Autodesk Fusion 360 part; units mm, degrees
(part 2 of 2)
extrude "Foro_M2_5_barretta_Destra_01" cut sketch "Schizzo2 (11)" along normal blind 3 bodies 12 in component "08_Barrette_removibili_M2_5_SG90_Destra"
ref_plane "Piano di lavoro3" through (63.5, 0, 0) normal (1, 0, 0) x (0, 1, 0) in component "08_Barrette_removibili_M2_5_SG90_Destra"
sketch "Schizzo3 (9)" plane through (63.5, 0, 0) normal (1, 0, 0) x (0, 0, -1) in component "08_Barrette_removibili_M2_5_SG90_Destra"
  line L0 (-68.4, 2.7) -> (-81.6, 2.7)
  line L1 (-81.6, 2.7) -> (-81.6, 13.5)
  line L2 (-81.6, 13.5) -> (-68.4, 13.5)
  line L3 (-68.4, 13.5) -> (-68.4, 2.7)
extrude "Estrusione_Barretta_Destra_02" add sketch "Schizzo3 (9)" along normal blind 3 separate body makes body 13 in component "08_Barrette_removibili_M2_5_SG90_Destra"
ref_plane "Piano di lavoro4" through (63.5, 0, 0) normal (1, 0, 0) x (0, 1, 0) in component "08_Barrette_removibili_M2_5_SG90_Destra"
sketch "Schizzo4 (8)" plane through (63.5, 0, 0) normal (1, 0, 0) x (0, 0, -1) in component "08_Barrette_removibili_M2_5_SG90_Destra"
  circle A0 centre (-75, 12.25) radius 1.35
extrude "Foro_M2_5_barretta_Destra_02" cut sketch "Schizzo4 (8)" along normal blind 3 bodies 13 in component "08_Barrette_removibili_M2_5_SG90_Destra"
ref_plane "Piano di lavoro1" through (0, 0, 73) normal (0, 0, 1) x (1, 0, 0) in component "09_Torretta_parte_mobile_elevazione"
sketch "Schizzo1 (13)" plane through (0, 0, 73) normal (0, 0, 1) x (1, 0, 0) in component "09_Torretta_parte_mobile_elevazione"
  line L0 (-34, -20) -> (34, -20)
  line L1 (34, -20) -> (34, 50)
  line L2 (34, 50) -> (-34, 50)
  line L3 (-34, 50) -> (-34, -20)
extrude "Estrusione_Piastra_culla_mobile" add sketch "Schizzo1 (13)" along normal blind 4 separate body makes body 14 in component "09_Torretta_parte_mobile_elevazione"
sketch "Schizzo2 (12)" plane through (0, 0, 73) normal (0, 0, 1) x (1, 0, 0) in component "09_Torretta_parte_mobile_elevazione"
  line L0 (-3, -17) -> (3, -17)
  line L1 (3, -17) -> (3, -13)
  line L2 (3, -13) -> (-3, -13)
  line L3 (-3, -13) -> (-3, -17)
extrude "Passaggio_6x4_connettore_cannone_sotto_culla" cut sketch "Schizzo2 (12)" along normal blind 4 bodies 14 in component "09_Torretta_parte_mobile_elevazione"
sketch "Schizzo3 (10)" plane through (0, 0, 73) normal (0, 0, 1) x (1, 0, 0) in component "09_Torretta_parte_mobile_elevazione"
  circle A0 centre (-20, -5) radius 1.75
extrude "Foro_fissaggio_PCB_cannone_01" cut sketch "Schizzo3 (10)" along normal blind 4 bodies 14 in component "09_Torretta_parte_mobile_elevazione"
sketch "Schizzo4 (9)" plane through (0, 0, 73) normal (0, 0, 1) x (1, 0, 0) in component "09_Torretta_parte_mobile_elevazione"
  line L0 (-17.1, -3.3257) -> (-20, -1.6514)
  line L1 (-20, -1.6514) -> (-22.9, -3.3257)
  line L2 (-22.9, -3.3257) -> (-22.9, -6.6743)
  line L3 (-22.9, -6.6743) -> (-20, -8.3486)
  line L4 (-20, -8.3486) -> (-17.1, -6.6743)
  line L5 (-17.1, -6.6743) -> (-17.1, -3.3257)
extrude "Sede_dado_M3_PCB_cannone_01" cut sketch "Schizzo4 (9)" along normal blind 2.6 bodies 14 in component "09_Torretta_parte_mobile_elevazione"
sketch "Schizzo5 (7)" plane through (0, 0, 73) normal (0, 0, 1) x (1, 0, 0) in component "09_Torretta_parte_mobile_elevazione"
  circle A0 centre (20, -5) radius 1.75
extrude "Foro_fissaggio_PCB_cannone_02" cut sketch "Schizzo5 (7)" along normal blind 4 bodies 14 in component "09_Torretta_parte_mobile_elevazione"
sketch "Schizzo6 (7)" plane through (0, 0, 73) normal (0, 0, 1) x (1, 0, 0) in component "09_Torretta_parte_mobile_elevazione"
  line L0 (22.9, -3.3257) -> (20, -1.6514)
  line L1 (20, -1.6514) -> (17.1, -3.3257)
  line L2 (17.1, -3.3257) -> (17.1, -6.6743)
  line L3 (17.1, -6.6743) -> (20, -8.3486)
  line L4 (20, -8.3486) -> (22.9, -6.6743)
  line L5 (22.9, -6.6743) -> (22.9, -3.3257)
extrude "Sede_dado_M3_PCB_cannone_02" cut sketch "Schizzo6 (7)" along normal blind 2.6 bodies 14 in component "09_Torretta_parte_mobile_elevazione"
sketch "Schizzo7 (7)" plane through (0, 0, 73) normal (0, 0, 1) x (1, 0, 0) in component "09_Torretta_parte_mobile_elevazione"
  circle A0 centre (-20, 35) radius 1.75
extrude "Foro_fissaggio_PCB_cannone_03" cut sketch "Schizzo7 (7)" along normal blind 4 bodies 14 in component "09_Torretta_parte_mobile_elevazione"
sketch "Schizzo8 (7)" plane through (0, 0, 73) normal (0, 0, 1) x (1, 0, 0) in component "09_Torretta_parte_mobile_elevazione"
  line L0 (-17.1, 36.6743) -> (-20, 38.3486)
  line L1 (-20, 38.3486) -> (-22.9, 36.6743)
  line L2 (-22.9, 36.6743) -> (-22.9, 33.3257)
  line L3 (-22.9, 33.3257) -> (-20, 31.6514)
  line L4 (-20, 31.6514) -> (-17.1, 33.3257)
  line L5 (-17.1, 33.3257) -> (-17.1, 36.6743)
extrude "Sede_dado_M3_PCB_cannone_03" cut sketch "Schizzo8 (7)" along normal blind 2.6 bodies 14 in component "09_Torretta_parte_mobile_elevazione"
sketch "Schizzo9 (7)" plane through (0, 0, 73) normal (0, 0, 1) x (1, 0, 0) in component "09_Torretta_parte_mobile_elevazione"
  circle A0 centre (20, 35) radius 1.75
extrude "Foro_fissaggio_PCB_cannone_04" cut sketch "Schizzo9 (7)" along normal blind 4 bodies 14 in component "09_Torretta_parte_mobile_elevazione"
sketch "Schizzo10 (7)" plane through (0, 0, 73) normal (0, 0, 1) x (1, 0, 0) in component "09_Torretta_parte_mobile_elevazione"
  line L0 (22.9, 36.6743) -> (20, 38.3486)
  line L1 (20, 38.3486) -> (17.1, 36.6743)
  line L2 (17.1, 36.6743) -> (17.1, 33.3257)
  line L3 (17.1, 33.3257) -> (20, 31.6514)
  line L4 (20, 31.6514) -> (22.9, 33.3257)
  line L5 (22.9, 33.3257) -> (22.9, 36.6743)
extrude "Sede_dado_M3_PCB_cannone_04" cut sketch "Schizzo10 (7)" along normal blind 2.6 bodies 14 in component "09_Torretta_parte_mobile_elevazione"
ref_plane "Piano di lavoro2" through (-34, 0, 0) normal (1, 0, 0) x (0, 1, 0) in component "09_Torretta_parte_mobile_elevazione"
sketch "Schizzo11 (7)" plane through (-34, 0, 0) normal (1, 0, 0) x (0, 0, -1) in component "09_Torretta_parte_mobile_elevazione"
  line L0 (-64, -12) -> (-86, -12)
  line L1 (-86, -12) -> (-86, 12)
  line L2 (-86, 12) -> (-64, 12)
  line L3 (-64, 12) -> (-64, -12)
extrude "Estrusione_Orecchio_mobile_Sinistra" add sketch "Schizzo11 (7)" along normal blind 4 bodies 14 in component "09_Torretta_parte_mobile_elevazione"
ref_plane "Piano di lavoro3" through (30, 0, 0) normal (1, 0, 0) x (0, 1, 0) in component "09_Torretta_parte_mobile_elevazione"
sketch "Schizzo12 (5)" plane through (30, 0, 0) normal (1, 0, 0) x (0, 0, -1) in component "09_Torretta_parte_mobile_elevazione"
  line L0 (-64, -12) -> (-86, -12)
  line L1 (-86, -12) -> (-86, 12)
  line L2 (-86, 12) -> (-64, 12)
  line L3 (-64, 12) -> (-64, -12)
extrude "Estrusione_Orecchio_mobile_Destra" add sketch "Schizzo12 (5)" along normal blind 4 bodies 14 in component "09_Torretta_parte_mobile_elevazione"
ref_plane "Piano di lavoro4" through (-40, 0, 0) normal (1, 0, 0) x (0, 1, 0) in component "09_Torretta_parte_mobile_elevazione"
sketch "Schizzo13 (4)" plane through (-40, 0, 0) normal (1, 0, 0) x (0, 0, -1) in component "09_Torretta_parte_mobile_elevazione"
  circle A0 centre (-75, 0) radius 3
extrude "Estrusione_Perno_servo_sinistro_coassiale" add sketch "Schizzo13 (4)" along normal blind 10 bodies 14 in component "09_Torretta_parte_mobile_elevazione"
ref_plane "Piano di lavoro5" through (30, 0, 0) normal (1, 0, 0) x (0, 1, 0) in component "09_Torretta_parte_mobile_elevazione"
sketch "Schizzo14 (4)" plane through (30, 0, 0) normal (1, 0, 0) x (0, 0, -1) in component "09_Torretta_parte_mobile_elevazione"
  circle A0 centre (-75, 0) radius 3
extrude "Estrusione_Perno_servo_destro_coassiale" add sketch "Schizzo14 (4)" along normal blind 10 bodies 14 in component "09_Torretta_parte_mobile_elevazione"
ref_plane "Piano di lavoro1" through (0, 0, 77) normal (0, 0, 1) x (1, 0, 0) in component "10_Modulo_cannone_reale_PCB_solenoide_canna"
sketch "Schizzo1 (14)" plane through (0, 0, 77) normal (0, 0, 1) x (1, 0, 0) in component "10_Modulo_cannone_reale_PCB_solenoide_canna"
  line L0 (-25, -10) -> (25, -10)
  line L1 (25, -10) -> (25, 40)
  line L2 (25, 40) -> (-25, 40)
  line L3 (-25, 40) -> (-25, -10)
extrude "Estrusione_PCB_modulo_cannone_50x50" add sketch "Schizzo1 (14)" along normal blind 2 separate body makes body 15 in component "10_Modulo_cannone_reale_PCB_solenoide_canna"
sketch "Schizzo2 (13)" plane through (0, 0, 77) normal (0, 0, 1) x (1, 0, 0) in component "10_Modulo_cannone_reale_PCB_solenoide_canna"
  circle A0 centre (-20, -5) radius 1.75
extrude "Foro_PCB_reale_01" cut sketch "Schizzo2 (13)" along normal blind 2 bodies 15 in component "10_Modulo_cannone_reale_PCB_solenoide_canna"
sketch "Schizzo3 (11)" plane through (0, 0, 77) normal (0, 0, 1) x (1, 0, 0) in component "10_Modulo_cannone_reale_PCB_solenoide_canna"
  circle A0 centre (20, -5) radius 1.75
extrude "Foro_PCB_reale_02" cut sketch "Schizzo3 (11)" along normal blind 2 bodies 15 in component "10_Modulo_cannone_reale_PCB_solenoide_canna"
sketch "Schizzo4 (10)" plane through (0, 0, 77) normal (0, 0, 1) x (1, 0, 0) in component "10_Modulo_cannone_reale_PCB_solenoide_canna"
  circle A0 centre (-20, 35) radius 1.75
extrude "Foro_PCB_reale_03" cut sketch "Schizzo4 (10)" along normal blind 2 bodies 15 in component "10_Modulo_cannone_reale_PCB_solenoide_canna"
sketch "Schizzo5 (8)" plane through (0, 0, 77) normal (0, 0, 1) x (1, 0, 0) in component "10_Modulo_cannone_reale_PCB_solenoide_canna"
  circle A0 centre (20, 35) radius 1.75
extrude "Foro_PCB_reale_04" cut sketch "Schizzo5 (8)" along normal blind 2 bodies 15 in component "10_Modulo_cannone_reale_PCB_solenoide_canna"
ref_plane "Piano di lavoro2" through (0, 0, 79) normal (0, 0, 1) x (1, 0, 0) in component "10_Modulo_cannone_reale_PCB_solenoide_canna"
sketch "Schizzo6 (8)" plane through (0, 0, 79) normal (0, 0, 1) x (1, 0, 0) in component "10_Modulo_cannone_reale_PCB_solenoide_canna"
  line L0 (-10, 2.5) -> (10, 2.5)
  line L1 (10, 2.5) -> (10, 27.5)
  line L2 (10, 27.5) -> (-10, 27.5)
  line L3 (-10, 27.5) -> (-10, 2.5)
extrude "Estrusione_Appoggio_solenoide_su_PCB" add sketch "Schizzo6 (8)" along normal blind 1 separate body makes body 16 in component "10_Modulo_cannone_reale_PCB_solenoide_canna"
ref_plane "Piano di lavoro3" through (0, 2.5, 0) normal (0, 1, 0) x (0, 0, 1) in component "10_Modulo_cannone_reale_PCB_solenoide_canna"
sketch "Schizzo7 (8)" plane through (0, 2.5, 0) normal (0, 1, 0) x (1, 0, 0) in component "10_Modulo_cannone_reale_PCB_solenoide_canna"
  circle A0 centre (0, -90) radius 10
extrude "Estrusione_Corpo_solenoide_riferimento" add sketch "Schizzo7 (8)" along normal blind 25 separate body makes body 17 in component "10_Modulo_cannone_reale_PCB_solenoide_canna"
ref_plane "Piano di lavoro4" through (0, 2.5, 0) normal (0, 1, 0) x (0, 0, 1) in component "10_Modulo_cannone_reale_PCB_solenoide_canna"
sketch "Schizzo8 (8)" plane through (0, 2.5, 0) normal (0, 1, 0) x (1, 0, 0) in component "10_Modulo_cannone_reale_PCB_solenoide_canna"
  circle A0 centre (0, -90) radius 5
extrude "Passaggio_canna_nel_solenoide" cut sketch "Schizzo8 (8)" along normal blind 25 bodies 17 in component "10_Modulo_cannone_reale_PCB_solenoide_canna"
ref_plane "Piano di lavoro5" through (0, 27.5, 0) normal (0, 1, 0) x (0, 0, 1) in component "10_Modulo_cannone_reale_PCB_solenoide_canna"
sketch "Schizzo9 (8)" plane through (0, 27.5, 0) normal (0, 1, 0) x (1, 0, 0) in component "10_Modulo_cannone_reale_PCB_solenoide_canna"
  circle A0 centre (0, -90) radius 5
extrude "Estrusione_Canna_tubolare_esterna" add sketch "Schizzo9 (8)" along normal blind 46 separate body makes body 18 in component "10_Modulo_cannone_reale_PCB_solenoide_canna"
ref_plane "Piano di lavoro6" through (0, 27.5, 0) normal (0, 1, 0) x (0, 0, 1) in component "10_Modulo_cannone_reale_PCB_solenoide_canna"
sketch "Schizzo10 (8)" plane through (0, 27.5, 0) normal (0, 1, 0) x (1, 0, 0) in component "10_Modulo_cannone_reale_PCB_solenoide_canna"
  circle A0 centre (0, -90) radius 4
extrude "Foro_interno_canna_tubolare" cut sketch "Schizzo10 (8)" along normal blind 46 bodies 18 in component "10_Modulo_cannone_reale_PCB_solenoide_canna"
ref_plane "Piano di lavoro1" through (0, -38, 0) normal (0, 1, 0) x (0, 0, 1) in component "11_Guscio_fisso_posteriore_torretta_removibile"
sketch "Schizzo1 (15)" plane through (0, -38, 0) normal (0, 1, 0) x (1, 0, 0) in component "11_Guscio_fisso_posteriore_torretta_removibile"
  line L0 (-43, -43) -> (43, -43)
  line L1 (43, -43) -> (43, -96)
  line L2 (43, -96) -> (-43, -96)
  line L3 (-43, -96) -> (-43, -43)
extrude "Estrusione_Parete_posteriore_guscio_torretta" add sketch "Schizzo1 (15)" along normal blind 2.5 separate body makes body 19 in component "11_Guscio_fisso_posteriore_torretta_removibile"
ref_plane "Piano di lavoro2" through (-43, 0, 0) normal (1, 0, 0) x (0, 1, 0) in component "11_Guscio_fisso_posteriore_torretta_removibile"
sketch "Schizzo2 (14)" plane through (-43, 0, 0) normal (1, 0, 0) x (0, 0, -1) in component "11_Guscio_fisso_posteriore_torretta_removibile"
  line L0 (-43, -38) -> (-96, -38)
  line L1 (-96, -38) -> (-96, -27.8)
  line L2 (-96, -27.8) -> (-43, -27.8)
  line L3 (-43, -27.8) -> (-43, -38)
extrude "Estrusione_Fianco_cofano_Sinistra" add sketch "Schizzo2 (14)" along normal blind 2.5 bodies 19 in component "11_Guscio_fisso_posteriore_torretta_removibile"
ref_plane "Piano di lavoro3" through (40.5, 0, 0) normal (1, 0, 0) x (0, 1, 0) in component "11_Guscio_fisso_posteriore_torretta_removibile"
sketch "Schizzo3 (12)" plane through (40.5, 0, 0) normal (1, 0, 0) x (0, 0, -1) in component "11_Guscio_fisso_posteriore_torretta_removibile"
  line L0 (-43, -38) -> (-96, -38)
  line L1 (-96, -38) -> (-96, -27.8)
  line L2 (-96, -27.8) -> (-43, -27.8)
  line L3 (-43, -27.8) -> (-43, -38)
extrude "Estrusione_Fianco_cofano_Destra" add sketch "Schizzo3 (12)" along normal blind 2.5 bodies 19 in component "11_Guscio_fisso_posteriore_torretta_removibile"
ref_plane "Piano di lavoro4" through (0, 0, 93.5) normal (0, 0, 1) x (1, 0, 0) in component "11_Guscio_fisso_posteriore_torretta_removibile"
sketch "Schizzo4 (11)" plane through (0, 0, 93.5) normal (0, 0, 1) x (1, 0, 0) in component "11_Guscio_fisso_posteriore_torretta_removibile"
  line L0 (-43, -38) -> (43, -38)
  line L1 (43, -38) -> (43, -27.8)
  line L2 (43, -27.8) -> (-43, -27.8)
  line L3 (-43, -27.8) -> (-43, -38)
extrude "Estrusione_Tetto_cofano_posteriore" add sketch "Schizzo4 (11)" along normal blind 2.5 bodies 19 in component "11_Guscio_fisso_posteriore_torretta_removibile"
ref_plane "Piano di lavoro5" through (-43, 0, 0) normal (1, 0, 0) x (0, 1, 0) in component "11_Guscio_fisso_posteriore_torretta_removibile"
sketch "Schizzo5 (9)" plane through (-43, 0, 0) normal (1, 0, 0) x (0, 0, -1) in component "11_Guscio_fisso_posteriore_torretta_removibile"
  circle A0 centre (-48, -30.3) radius 1.35
extrude "Foro_M2_5_cofano_Sinistra_01" cut sketch "Schizzo5 (9)" along normal blind 2.5 bodies 19 in component "11_Guscio_fisso_posteriore_torretta_removibile"
ref_plane "Piano di lavoro22" through (-40, 0, 0) normal (1, 0, 0) x (0, 1, 0) in component "04_Torretta_parte_fissa_azimut"
sketch "Schizzo27" plane through (-40, 0, 0) normal (1, 0, 0) x (0, 0, -1) in component "04_Torretta_parte_fissa_azimut"
  circle A0 centre (-48, -30.3) radius 1.1
extrude "Preforo_M2_5_cofano_telaio_Sinistra_01" cut sketch "Schizzo27" along normal blind 4 bodies 7 in component "04_Torretta_parte_fissa_azimut"
ref_plane "Piano di lavoro6" through (-43, 0, 0) normal (1, 0, 0) x (0, 1, 0) in component "11_Guscio_fisso_posteriore_torretta_removibile"
sketch "Schizzo6 (9)" plane through (-43, 0, 0) normal (1, 0, 0) x (0, 0, -1) in component "11_Guscio_fisso_posteriore_torretta_removibile"
  circle A0 centre (-88, -30.3) radius 1.35
extrude "Foro_M2_5_cofano_Sinistra_02" cut sketch "Schizzo6 (9)" along normal blind 2.5 bodies 19 in component "11_Guscio_fisso_posteriore_torretta_removibile"
ref_plane "Piano di lavoro23" through (-40, 0, 0) normal (1, 0, 0) x (0, 1, 0) in component "04_Torretta_parte_fissa_azimut"
sketch "Schizzo28" plane through (-40, 0, 0) normal (1, 0, 0) x (0, 0, -1) in component "04_Torretta_parte_fissa_azimut"
  circle A0 centre (-88, -30.3) radius 1.1
extrude "Preforo_M2_5_cofano_telaio_Sinistra_02" cut sketch "Schizzo28" along normal blind 4 bodies 7 in component "04_Torretta_parte_fissa_azimut"
ref_plane "Piano di lavoro7" through (40.5, 0, 0) normal (1, 0, 0) x (0, 1, 0) in component "11_Guscio_fisso_posteriore_torretta_removibile"
sketch "Schizzo7 (9)" plane through (40.5, 0, 0) normal (1, 0, 0) x (0, 0, -1) in component "11_Guscio_fisso_posteriore_torretta_removibile"
  circle A0 centre (-48, -30.3) radius 1.35
extrude "Foro_M2_5_cofano_Destra_01" cut sketch "Schizzo7 (9)" along normal blind 2.5 bodies 19 in component "11_Guscio_fisso_posteriore_torretta_removibile"
ref_plane "Piano di lavoro24" through (36, 0, 0) normal (1, 0, 0) x (0, 1, 0) in component "04_Torretta_parte_fissa_azimut"
sketch "Schizzo29" plane through (36, 0, 0) normal (1, 0, 0) x (0, 0, -1) in component "04_Torretta_parte_fissa_azimut"
  circle A0 centre (-48, -30.3) radius 1.1
extrude "Preforo_M2_5_cofano_telaio_Destra_01" cut sketch "Schizzo29" along normal blind 4 bodies 7 in component "04_Torretta_parte_fissa_azimut"
ref_plane "Piano di lavoro8" through (40.5, 0, 0) normal (1, 0, 0) x (0, 1, 0) in component "11_Guscio_fisso_posteriore_torretta_removibile"
sketch "Schizzo8 (9)" plane through (40.5, 0, 0) normal (1, 0, 0) x (0, 0, -1) in component "11_Guscio_fisso_posteriore_torretta_removibile"
  circle A0 centre (-88, -30.3) radius 1.35
extrude "Foro_M2_5_cofano_Destra_02" cut sketch "Schizzo8 (9)" along normal blind 2.5 bodies 19 in component "11_Guscio_fisso_posteriore_torretta_removibile"
ref_plane "Piano di lavoro25" through (36, 0, 0) normal (1, 0, 0) x (0, 1, 0) in component "04_Torretta_parte_fissa_azimut"
sketch "Schizzo30" plane through (36, 0, 0) normal (1, 0, 0) x (0, 0, -1) in component "04_Torretta_parte_fissa_azimut"
  circle A0 centre (-88, -30.3) radius 1.1
extrude "Preforo_M2_5_cofano_telaio_Destra_02" cut sketch "Schizzo30" along normal blind 4 bodies 7 in component "04_Torretta_parte_fissa_azimut"
ref_plane "Piano di lavoro1" through (-69.5, 0, 0) normal (1, 0, 0) x (0, 1, 0) in component "12_Carter_SG90_Sinistro_removibile"
sketch "Schizzo1 (16)" plane through (-69.5, 0, 0) normal (1, 0, 0) x (0, 0, -1) in component "12_Carter_SG90_Sinistro_removibile"
  line L0 (-65.4, -27.8) -> (-87.1, -27.8)
  line L1 (-87.1, -27.8) -> (-87.1, 16.5)
  line L2 (-87.1, 16.5) -> (-65.4, 16.5)
  line L3 (-65.4, 16.5) -> (-65.4, -27.8)
extrude "Estrusione_Parete_esterna_carter_Sinistro" add sketch "Schizzo1 (16)" along normal blind 2.5 separate body makes body 20 in component "12_Carter_SG90_Sinistro_removibile"
ref_plane "Piano di lavoro2" through (0, -27.8, 0) normal (0, 1, 0) x (0, 0, 1) in component "12_Carter_SG90_Sinistro_removibile"
sketch "Schizzo2 (15)" plane through (0, -27.8, 0) normal (0, 1, 0) x (1, 0, 0) in component "12_Carter_SG90_Sinistro_removibile"
  line L0 (-69.5, -65.4) -> (-40.5, -65.4)
  line L1 (-40.5, -65.4) -> (-40.5, -87.1)
  line L2 (-40.5, -87.1) -> (-69.5, -87.1)
  line L3 (-69.5, -87.1) -> (-69.5, -65.4)
extrude "Estrusione_Parete_Posteriore_carter_Sinistro" add sketch "Schizzo2 (15)" along normal blind 2.5 bodies 20 in component "12_Carter_SG90_Sinistro_removibile"
ref_plane "Piano di lavoro3" through (0, 14, 0) normal (0, 1, 0) x (0, 0, 1) in component "12_Carter_SG90_Sinistro_removibile"
sketch "Schizzo3 (13)" plane through (0, 14, 0) normal (0, 1, 0) x (1, 0, 0) in component "12_Carter_SG90_Sinistro_removibile"
  line L0 (-69.5, -65.4) -> (-40.5, -65.4)
  line L1 (-40.5, -65.4) -> (-40.5, -87.1)
  line L2 (-40.5, -87.1) -> (-69.5, -87.1)
  line L3 (-69.5, -87.1) -> (-69.5, -65.4)
extrude "Estrusione_Parete_Anteriore_carter_Sinistro" add sketch "Schizzo3 (13)" along normal blind 2.5 bodies 20 in component "12_Carter_SG90_Sinistro_removibile"
ref_plane "Piano di lavoro4" through (0, 0, 84.6) normal (0, 0, 1) x (1, 0, 0) in component "12_Carter_SG90_Sinistro_removibile"
sketch "Schizzo4 (12)" plane through (0, 0, 84.6) normal (0, 0, 1) x (1, 0, 0) in component "12_Carter_SG90_Sinistro_removibile"
  line L0 (-69.5, -27.8) -> (-40.5, -27.8)
  line L1 (-40.5, -27.8) -> (-40.5, 16.5)
  line L2 (-40.5, 16.5) -> (-69.5, 16.5)
  line L3 (-69.5, 16.5) -> (-69.5, -27.8)
extrude "Estrusione_Tetto_carter_Sinistro" add sketch "Schizzo4 (12)" along normal blind 2.5 bodies 20 in component "12_Carter_SG90_Sinistro_removibile"
ref_plane "Piano di lavoro5" through (-69.5, 0, 0) normal (1, 0, 0) x (0, 1, 0) in component "12_Carter_SG90_Sinistro_removibile"
sketch "Schizzo5 (10)" plane through (-69.5, 0, 0) normal (1, 0, 0) x (0, 0, -1) in component "12_Carter_SG90_Sinistro_removibile"
  circle A0 centre (-75, -23.55) radius 1.35
extrude "Foro_M2_5_carter_Sinistro_01" cut sketch "Schizzo5 (10)" along normal blind 2.5 bodies 20 in component "12_Carter_SG90_Sinistro_removibile"
ref_plane "Piano di lavoro6" through (-69.5, 0, 0) normal (1, 0, 0) x (0, 1, 0) in component "12_Carter_SG90_Sinistro_removibile"
sketch "Schizzo6 (10)" plane through (-69.5, 0, 0) normal (1, 0, 0) x (0, 0, -1) in component "12_Carter_SG90_Sinistro_removibile"
  circle A0 centre (-75, 12.25) radius 1.35
extrude "Foro_M2_5_carter_Sinistro_02" cut sketch "Schizzo6 (10)" along normal blind 2.5 bodies 20 in component "12_Carter_SG90_Sinistro_removibile"
ref_plane "Piano di lavoro1" through (67, 0, 0) normal (1, 0, 0) x (0, 1, 0) in component "13_Carter_SG90_Destro_removibile"
sketch "Schizzo1 (17)" plane through (67, 0, 0) normal (1, 0, 0) x (0, 0, -1) in component "13_Carter_SG90_Destro_removibile"
  line L0 (-65.4, -27.8) -> (-87.1, -27.8)
  line L1 (-87.1, -27.8) -> (-87.1, 16.5)
  line L2 (-87.1, 16.5) -> (-65.4, 16.5)
  line L3 (-65.4, 16.5) -> (-65.4, -27.8)
extrude "Estrusione_Parete_esterna_carter_Destro" add sketch "Schizzo1 (17)" along normal blind 2.5 separate body makes body 21 in component "13_Carter_SG90_Destro_removibile"
ref_plane "Piano di lavoro2" through (0, -27.8, 0) normal (0, 1, 0) x (0, 0, 1) in component "13_Carter_SG90_Destro_removibile"
sketch "Schizzo2 (16)" plane through (0, -27.8, 0) normal (0, 1, 0) x (1, 0, 0) in component "13_Carter_SG90_Destro_removibile"
  line L0 (40.5, -65.4) -> (69.5, -65.4)
  line L1 (69.5, -65.4) -> (69.5, -87.1)
  line L2 (69.5, -87.1) -> (40.5, -87.1)
  line L3 (40.5, -87.1) -> (40.5, -65.4)
extrude "Estrusione_Parete_Posteriore_carter_Destro" add sketch "Schizzo2 (16)" along normal blind 2.5 bodies 21 in component "13_Carter_SG90_Destro_removibile"
ref_plane "Piano di lavoro3" through (0, 14, 0) normal (0, 1, 0) x (0, 0, 1) in component "13_Carter_SG90_Destro_removibile"
sketch "Schizzo3 (14)" plane through (0, 14, 0) normal (0, 1, 0) x (1, 0, 0) in component "13_Carter_SG90_Destro_removibile"
  line L0 (40.5, -65.4) -> (69.5, -65.4)
  line L1 (69.5, -65.4) -> (69.5, -87.1)
  line L2 (69.5, -87.1) -> (40.5, -87.1)
  line L3 (40.5, -87.1) -> (40.5, -65.4)
extrude "Estrusione_Parete_Anteriore_carter_Destro" add sketch "Schizzo3 (14)" along normal blind 2.5 bodies 21 in component "13_Carter_SG90_Destro_removibile"
ref_plane "Piano di lavoro4" through (0, 0, 84.6) normal (0, 0, 1) x (1, 0, 0) in component "13_Carter_SG90_Destro_removibile"
sketch "Schizzo4 (13)" plane through (0, 0, 84.6) normal (0, 0, 1) x (1, 0, 0) in component "13_Carter_SG90_Destro_removibile"
  line L0 (40.5, -27.8) -> (69.5, -27.8)
  line L1 (69.5, -27.8) -> (69.5, 16.5)
  line L2 (69.5, 16.5) -> (40.5, 16.5)
  line L3 (40.5, 16.5) -> (40.5, -27.8)
extrude "Estrusione_Tetto_carter_Destro" add sketch "Schizzo4 (13)" along normal blind 2.5 bodies 21 in component "13_Carter_SG90_Destro_removibile"
ref_plane "Piano di lavoro5" through (67, 0, 0) normal (1, 0, 0) x (0, 1, 0) in component "13_Carter_SG90_Destro_removibile"
sketch "Schizzo5 (11)" plane through (67, 0, 0) normal (1, 0, 0) x (0, 0, -1) in component "13_Carter_SG90_Destro_removibile"
  circle A0 centre (-75, -23.55) radius 1.35
extrude "Foro_M2_5_carter_Destro_01" cut sketch "Schizzo5 (11)" along normal blind 2.5 bodies 21 in component "13_Carter_SG90_Destro_removibile"
ref_plane "Piano di lavoro6" through (67, 0, 0) normal (1, 0, 0) x (0, 1, 0) in component "13_Carter_SG90_Destro_removibile"
sketch "Schizzo6 (11)" plane through (67, 0, 0) normal (1, 0, 0) x (0, 0, -1) in component "13_Carter_SG90_Destro_removibile"
  circle A0 centre (-75, 12.25) radius 1.35
extrude "Foro_M2_5_carter_Destro_02" cut sketch "Schizzo6 (11)" along normal blind 2.5 bodies 21 in component "13_Carter_SG90_Destro_removibile"
ref_plane "Piano di lavoro1" through (0, 0, 77) normal (0, 0, 1) x (1, 0, 0) in component "14_Guscio_mobile_cannone_removibile"
sketch "Schizzo1 (18)" plane through (0, 0, 77) normal (0, 0, 1) x (1, 0, 0) in component "14_Guscio_mobile_cannone_removibile"
  line L0 (-28, -13) -> (-25.5, -13)
  line L1 (-25.5, -13) -> (-25.5, 43)
  line L2 (-25.5, 43) -> (-28, 43)
  line L3 (-28, 43) -> (-28, -13)
extrude "Estrusione_Parete_mobile_Ovest" add sketch "Schizzo1 (18)" along normal blind 26 separate body makes body 22 in component "14_Guscio_mobile_cannone_removibile"
sketch "Schizzo2 (17)" plane through (0, 0, 77) normal (0, 0, 1) x (1, 0, 0) in component "14_Guscio_mobile_cannone_removibile"
  line L0 (-28, -13) -> (28, -13)
  line L1 (28, -13) -> (28, -10.5)
  line L2 (28, -10.5) -> (-28, -10.5)
  line L3 (-28, -10.5) -> (-28, -13)
extrude "Estrusione_Parete_mobile_Posteriore" add sketch "Schizzo2 (17)" along normal blind 26 bodies 22 in component "14_Guscio_mobile_cannone_removibile"
sketch "Schizzo3 (15)" plane through (0, 0, 77) normal (0, 0, 1) x (1, 0, 0) in component "14_Guscio_mobile_cannone_removibile"
  line L0 (25.5, -13) -> (28, -13)
  line L1 (28, -13) -> (28, 43)
  line L2 (28, 43) -> (25.5, 43)
  line L3 (25.5, 43) -> (25.5, -13)
extrude "Estrusione_Parete_mobile_Est" add sketch "Schizzo3 (15)" along normal blind 26 bodies 22 in component "14_Guscio_mobile_cannone_removibile"
sketch "Schizzo4 (14)" plane through (0, 0, 77) normal (0, 0, 1) x (1, 0, 0) in component "14_Guscio_mobile_cannone_removibile"
  line L0 (-28, 40.5) -> (28, 40.5)
  line L1 (28, 40.5) -> (28, 43)
  line L2 (28, 43) -> (-28, 43)
  line L3 (-28, 43) -> (-28, 40.5)
extrude "Estrusione_Parete_mobile_Anteriore" add sketch "Schizzo4 (14)" along normal blind 26 bodies 22 in component "14_Guscio_mobile_cannone_removibile"
ref_plane "Piano di lavoro2" through (0, 0, 100.5) normal (0, 0, 1) x (1, 0, 0) in component "14_Guscio_mobile_cannone_removibile"
sketch "Schizzo5 (12)" plane through (0, 0, 100.5) normal (0, 0, 1) x (1, 0, 0) in component "14_Guscio_mobile_cannone_removibile"
  line L0 (-28, -13) -> (28, -13)
  line L1 (28, -13) -> (28, 43)
  line L2 (28, 43) -> (-28, 43)
  line L3 (-28, 43) -> (-28, -13)
extrude "Estrusione_Tetto_guscio_mobile_cannone" add sketch "Schizzo5 (12)" along normal blind 2.5 bodies 22 in component "14_Guscio_mobile_cannone_removibile"
ref_plane "Piano di lavoro3" through (0, 40.5, 0) normal (0, 1, 0) x (0, 0, 1) in component "14_Guscio_mobile_cannone_removibile"
sketch "Schizzo6 (12)" plane through (0, 40.5, 0) normal (0, 1, 0) x (1, 0, 0) in component "14_Guscio_mobile_cannone_removibile"
  circle A0 centre (0, -90) radius 5.5
extrude "Passaggio_canna_guscio_mobile_diametro_11" cut sketch "Schizzo6 (12)" along normal blind 2.5 bodies 18 makes body 23 at (4.9752, 36.1667, 89.5022) in component "10_Modulo_cannone_reale_PCB_solenoide_canna"
extrude "Estrusione6" cut sketch "Schizzo6 (12)" along normal blind 2.5 bodies 22 in component "14_Guscio_mobile_cannone_removibile"
ref_plane "Piano di lavoro4" through (0, 40.5, 0) normal (0, 1, 0) x (0, 0, 1) in component "14_Guscio_mobile_cannone_removibile"
sketch "Schizzo7 (10)" plane through (0, 40.5, 0) normal (0, 1, 0) x (1, 0, 0) in component "14_Guscio_mobile_cannone_removibile"
  line L0 (-5.5, -77) -> (5.5, -77)
  line L1 (5.5, -77) -> (5.5, -90)
  line L2 (5.5, -90) -> (-5.5, -90)
  line L3 (-5.5, -90) -> (-5.5, -77)
extrude "Cava_U_inferiore_smontaggio_guscio_mobile" cut sketch "Schizzo7 (10)" along normal blind 2.5 bodies 22 in component "14_Guscio_mobile_cannone_removibile"
ref_plane "Piano di lavoro5" through (0, -13, 0) normal (0, 1, 0) x (0, 0, 1) in component "14_Guscio_mobile_cannone_removibile"
sketch "Schizzo8 (10)" plane through (0, -13, 0) normal (0, 1, 0) x (1, 0, 0) in component "14_Guscio_mobile_cannone_removibile"
  line L0 (-3, -77) -> (3, -77)
  line L1 (3, -77) -> (3, -81)
  line L2 (3, -81) -> (-3, -81)
  line L3 (-3, -81) -> (-3, -77)
extrude "Tacca_posteriore_cavo_cannone_aperta_inferiormente" cut sketch "Schizzo8 (10)" along normal blind 2.5 bodies 22 in component "14_Guscio_mobile_cannone_removibile"
ref_plane "Piano di lavoro6" through (0, 0, 79) normal (0, 0, 1) x (1, 0, 0) in component "14_Guscio_mobile_cannone_removibile"
sketch "Schizzo9 (9)" plane through (0, 0, 79) normal (0, 0, 1) x (1, 0, 0) in component "14_Guscio_mobile_cannone_removibile"
  circle A0 centre (-20, -5) radius 5
extrude "Estrusione_Colonna_M3_guscio_mobile_01" add sketch "Schizzo9 (9)" along normal blind 21.7 bodies 22 in component "14_Guscio_mobile_cannone_removibile"
sketch "Schizzo10 (9)" plane through (0, 0, 79) normal (0, 0, 1) x (1, 0, 0) in component "14_Guscio_mobile_cannone_removibile"
  circle A0 centre (-20, -5) radius 1.75
extrude "Foro_M3_guscio_mobile_01" cut sketch "Schizzo10 (9)" along normal blind 24 bodies 22 in component "14_Guscio_mobile_cannone_removibile"
sketch "Schizzo11 (8)" plane through (0, 0, 79) normal (0, 0, 1) x (1, 0, 0) in component "14_Guscio_mobile_cannone_removibile"
  circle A0 centre (20, -5) radius 5
extrude "Estrusione_Colonna_M3_guscio_mobile_02" add sketch "Schizzo11 (8)" along normal blind 21.7 bodies 22 in component "14_Guscio_mobile_cannone_removibile"
sketch "Schizzo12 (6)" plane through (0, 0, 79) normal (0, 0, 1) x (1, 0, 0) in component "14_Guscio_mobile_cannone_removibile"
  circle A0 centre (20, -5) radius 1.75
extrude "Foro_M3_guscio_mobile_02" cut sketch "Schizzo12 (6)" along normal blind 24 bodies 22 in component "14_Guscio_mobile_cannone_removibile"
sketch "Schizzo13 (5)" plane through (0, 0, 79) normal (0, 0, 1) x (1, 0, 0) in component "14_Guscio_mobile_cannone_removibile"
  circle A0 centre (-20, 35) radius 5
extrude "Estrusione_Colonna_M3_guscio_mobile_03" add sketch "Schizzo13 (5)" along normal blind 21.7 bodies 22 in component "14_Guscio_mobile_cannone_removibile"
sketch "Schizzo14 (5)" plane through (0, 0, 79) normal (0, 0, 1) x (1, 0, 0) in component "14_Guscio_mobile_cannone_removibile"
  circle A0 centre (-20, 35) radius 1.75
extrude "Foro_M3_guscio_mobile_03" cut sketch "Schizzo14 (5)" along normal blind 24 bodies 22 in component "14_Guscio_mobile_cannone_removibile"
sketch "Schizzo15 (4)" plane through (0, 0, 79) normal (0, 0, 1) x (1, 0, 0) in component "14_Guscio_mobile_cannone_removibile"
  circle A0 centre (20, 35) radius 5
extrude "Estrusione_Colonna_M3_guscio_mobile_04" add sketch "Schizzo15 (4)" along normal blind 21.7 bodies 22 in component "14_Guscio_mobile_cannone_removibile"
sketch "Schizzo16 (4)" plane through (0, 0, 79) normal (0, 0, 1) x (1, 0, 0) in component "14_Guscio_mobile_cannone_removibile"
  circle A0 centre (20, 35) radius 1.75
extrude "Foro_M3_guscio_mobile_04" cut sketch "Schizzo16 (4)" along normal blind 24 bodies 22 in component "14_Guscio_mobile_cannone_removibile"
sketch "Schizzo1 (19)" plane through (0, 0, 0) normal (0, 1, 0) x (1, 0, 0) in component "06_Sottoassieme_coperchio_stepper_torretta"
  line L0 (0, -20) -> (0, 20)
ref_plane "Piano di lavoro1" through (0, 0, 75) normal (0, 0, 1) x (1, 0, 0) in component "06_Sottoassieme_coperchio_stepper_torretta"
sketch "Schizzo2 (18)" plane through (0, 0, 75) normal (0, 0, 1) x (1, 0, 0) in component "06_Sottoassieme_coperchio_stepper_torretta"
  line L0 (-20, 0) -> (20, 0)
component "01_Piano_inferiore_colonnine_M3_supporto_batteria_integrato" placed x (1, 0, 0) y (0, 1, 0) z (0, 0, 1) at (0, 0, 0)
component "02_Piano_superiore" placed x (1, 0, 0) y (0, 1, 0) z (0, 0, 1) at (0, 0, 0)
component "03_Guscio_laterale_continuo_carro" placed x (1, 0, 0) y (0, 1, 0) z (0, 0, 1) at (0, 0, 0)
component "05_Arduino_UNO_R4_WiFi_RIFERIMENTO_XY_quota_Z_da_definire" placed x (1, 0, 0) y (0, 1, 0) z (0, 0, 1) at (33.33, 45.71, 3)
component "06_Sottoassieme_coperchio_stepper_torretta" placed x (1, 0, 0) y (0, 1, 0) z (0, 0, 1) at (0, 0, 46)
component "01_Tetto_elettronica_removibile" placed x (1, 0, 0) y (0, 1, 0) z (0, 0, 1) at (0, 0, 0) in component "06_Sottoassieme_coperchio_stepper_torretta"
component "02_Stepper_28BYJ48_riferimento" placed x (1, 0, 0) y (0, 1, 0) z (0, 0, 1) at (0, 0, 0) in component "06_Sottoassieme_coperchio_stepper_torretta"
component "03_Adattatore_rotante_stepper" placed x (1, 0, 0) y (0, 1, 0) z (0, 0, 1) at (0, 0, 0) in component "06_Sottoassieme_coperchio_stepper_torretta"
component "04_Torretta_parte_fissa_azimut" placed x (1, 0, 0) y (0, 1, 0) z (0, 0, 1) at (0, 0, 0) in component "06_Sottoassieme_coperchio_stepper_torretta"
component "05_Servo_TowerPro_SG90_Sinistro_riferimento" placed x (1, 0, 0) y (0, 1, 0) z (0, 0, 1) at (0, 0, 0) in component "06_Sottoassieme_coperchio_stepper_torretta"
component "06_Servo_TowerPro_SG90_Destro_riferimento" placed x (1, 0, 0) y (0, 1, 0) z (0, 0, 1) at (0, 0, 0) in component "06_Sottoassieme_coperchio_stepper_torretta"
component "07_Barrette_removibili_M2_5_SG90_Sinistra" placed x (1, 0, 0) y (0, 1, 0) z (0, 0, 1) at (0, 0, 0) in component "06_Sottoassieme_coperchio_stepper_torretta"
component "08_Barrette_removibili_M2_5_SG90_Destra" placed x (1, 0, 0) y (0, 1, 0) z (0, 0, 1) at (0, 0, 0) in component "06_Sottoassieme_coperchio_stepper_torretta"
component "09_Torretta_parte_mobile_elevazione" placed x (1, 0, 0) y (0, 1, 0) z (0, 0, 1) at (0, 0, 0) in component "06_Sottoassieme_coperchio_stepper_torretta"
component "10_Modulo_cannone_reale_PCB_solenoide_canna" placed x (1, 0, 0) y (0, 1, 0) z (0, 0, 1) at (0, 0, 0) in component "06_Sottoassieme_coperchio_stepper_torretta"
component "11_Guscio_fisso_posteriore_torretta_removibile" placed x (1, 0, 0) y (0, 1, 0) z (0, 0, 1) at (0, 0, 0) in component "06_Sottoassieme_coperchio_stepper_torretta"
component "12_Carter_SG90_Sinistro_removibile" placed x (1, 0, 0) y (0, 1, 0) z (0, 0, 1) at (0, 0, 0) in component "06_Sottoassieme_coperchio_stepper_torretta"
component "13_Carter_SG90_Destro_removibile" placed x (1, 0, 0) y (0, 1, 0) z (0, 0, 1) at (0, 0, 0) in component "06_Sottoassieme_coperchio_stepper_torretta"
component "14_Guscio_mobile_cannone_removibile" placed x (1, 0, 0) y (0, 1, 0) z (0, 0, 1) at (0, 0, 0) in component "06_Sottoassieme_coperchio_stepper_torretta"
equation "piano_inf_lunghezza = 170.0 mm" comment "Piano inferiore"
equation "piano_inf_larghezza = 160.0 mm" comment "Piano inferiore"
equation "piano_inf_spessore = 3.0 mm" comment "Piano inferiore"
equation "d4 = piano_inf_spessore"
equation "distanza_piani = 40.0 mm" comment "Luce libera fra i piani"
equation "piano_sup_lunghezza = 170.0 mm" comment "Piano superiore"
equation "piano_sup_larghezza = 160.0 mm" comment "Piano superiore"
equation "piano_sup_spessore = 3.0 mm" comment "Piano superiore"
equation "colonnina_diametro = 10.0 mm" comment "Colonnine base"
equation "foro_vite_M3 = 3.2 mm" comment "Gioco vite M3"
equation "colonnina_offset_bordo = 12.0 mm" comment "Centro colonnina dal bordo"
equation "dado_M3_chiave = 5.8 mm" comment "Sede esagonale dado M3"
equation "dado_M3_profondita = 2.6 mm" comment "Profondita sede dado M3"
equation "d15 = piano_inf_spessore + distanza_piani"
equation "d17 = piano_sup_spessore"
equation "d19 = piano_inf_spessore"
equation "d21 = piano_inf_spessore + distanza_piani - dado_M3_profondita"
equation "asola_fascetta_lunghezza = 10.0 mm" comment "Asola fascetta, asse Est-Ovest"
equation "asola_fascetta_larghezza = 5.0 mm" comment "Asola fascetta, asse Sud-Nord"
equation "d25 = piano_inf_spessore"
equation "d27 = piano_inf_spessore"
equation "d29 = piano_inf_spessore"
equation "d31 = piano_inf_spessore"
equation "d33 = piano_sup_spessore"
equation "d35 = distanza_piani"
equation "d37 = piano_inf_spessore + distanza_piani"
equation "d39 = dado_M3_profondita"
equation "d41 = piano_sup_spessore"
equation "d43 = distanza_piani"
equation "d45 = piano_inf_spessore + distanza_piani"
equation "d47 = dado_M3_profondita"
equation "d49 = piano_sup_spessore"
equation "d51 = distanza_piani"
equation "d53 = piano_inf_spessore + distanza_piani"
equation "d55 = dado_M3_profondita"
equation "d57 = piano_sup_spessore"
equation "d59 = distanza_piani"
equation "d61 = piano_inf_spessore + distanza_piani"
equation "d63 = dado_M3_profondita"
equation "apertura_arduino_larghezza = 25.0 mm" comment "Apertura superiore sopra Arduino"
equation "apertura_arduino_lunghezza = 25.0 mm" comment "Apertura superiore sopra Arduino"
equation "apertura_arduino_centro_x = 33.33 mm" comment "Centro Est-Ovest apertura Arduino"
equation "apertura_arduino_centro_y = 45.71 mm" comment "Centro Sud-Nord apertura Arduino"
equation "apertura_pacco_batteria_larghezza = 33.0 mm" comment "Apertura superiore pacco batteria PCB cannone"
equation "apertura_pacco_batteria_lunghezza = 60.0 mm" comment "Apertura superiore pacco batteria PCB cannone"
equation "apertura_pacco_batteria_centro_x = -52.5 mm" comment "Centro Est-Ovest apertura pacco batteria PCB cannone"
equation "apertura_pacco_batteria_centro_y = -15.0 mm" comment "Centro Sud-Nord apertura pacco batteria PCB cannone"
equation "d73 = piano_sup_spessore"
equation "d75 = piano_sup_spessore"
equation "foro_piano_superiore_M2_5_guscio = 2.7 mm" comment "Quattro viti M2.5x8 per trattenere il guscio inferiore"
equation "d78 = piano_sup_spessore"
equation "d80 = piano_sup_spessore"
equation "d82 = piano_sup_spessore"
equation "d84 = piano_sup_spessore"
equation "batt_vano_lunghezza = 95.0 mm" comment "Vano batteria"
equation "batt_vano_larghezza = 40.0 mm" comment "Vano batteria"
equation "batt_esterno_lunghezza = 100.0 mm" comment "Supporto batteria"
equation "batt_esterno_larghezza = 45.0 mm" comment "Supporto batteria"
equation "batt_parete_spessore = 2.5 mm" comment "Pareti laterali"
equation "batt_parete_altezza = 17.0 mm" comment "Pareti laterali"
equation "batt_apertura_cavi = 10.0 mm" comment "Passaggio cavi"
equation "d93 = piano_inf_spessore"
equation "d95 = batt_parete_altezza"
equation "d97 = batt_parete_altezza"
equation "d99 = batt_parete_altezza"
equation "d101 = batt_parete_altezza"
equation "guscio_carro_larghezza_interna = 161.0 mm" comment "Vano interno guscio carro"
equation "guscio_carro_lunghezza_interna = 171.0 mm" comment "Vano interno guscio carro"
equation "guscio_carro_larghezza_esterna = 166.0 mm" comment "Ingombro esterno guscio carro"
equation "guscio_carro_lunghezza_esterna = 176.0 mm" comment "Ingombro esterno guscio carro"
equation "guscio_carro_parete = 2.5 mm" comment "Pareti guscio removibile"
equation "guscio_carro_altezza_inferiore = 46.0 mm" comment "Da piano inferiore a sommità piano superiore"
equation "guscio_carro_gioco_lato = 0.5 mm" comment "Gioco per lato rispetto ai piani"
equation "guscio_carro_altezza_laterale_continua = 76.0 mm" comment "Parete unica senza giunzione intermedia"
equation "guscio_linguetta_M2_5_spessore = 5.0 mm" comment "Fissaggio guscio sotto il piano superiore"
equation "guscio_linguetta_M2_5_span = 14.0 mm" comment "Fissaggio guscio sotto il piano superiore"
equation "guscio_linguetta_M2_5_profondita = 13.0 mm" comment "Fissaggio guscio sotto il piano superiore"
equation "guscio_linguetta_M2_5_preforo = 2.2 mm" comment "Preforo per M2.5x8"
equation "d115 = guscio_carro_altezza_laterale_continua"
equation "d117 = guscio_carro_altezza_laterale_continua"
equation "d119 = guscio_carro_altezza_laterale_continua"
equation "d121 = guscio_carro_altezza_laterale_continua"
equation "arduino_r4_lunghezza = 68.58 mm" comment "Profilo ufficiale Arduino UNO R4 WiFi"
equation "arduino_r4_larghezza = 53.34 mm" comment "Profilo ufficiale Arduino UNO R4 WiFi"
equation "arduino_r4_spessore_pcb = 1.0 mm" comment "Spessore PCB ufficiale; quota Z di montaggio non ancora definita"
equation "arduino_r4_rotazione = 90.0 deg" comment "Jack DC orientato verso Sud"
equation "arduino_r4_centro_x = 33.33 mm" comment "Posizione planimetrica Arduino"
equation "arduino_r4_centro_y = 45.71 mm" comment "Posizione planimetrica Arduino"
equation "cop_lunghezza = 176.0 mm" comment "Ingombro coperchio"
equation "cop_larghezza = 166.0 mm" comment "Ingombro coperchio"
equation "cop_parete_altezza = 30.0 mm" comment "Quota locale del tetto removibile"
equation "cop_tetto_spessore = 3.0 mm" comment "Coperchio elettronica"
equation "cop_boss_M3_diametro = 10.0 mm" comment "Accesso vite M3 dal tetto alle colonnine"
equation "cop_canale_fondo_raggio_interno = 19.0 mm" comment "Fondo liscio pista cavi tipo clock-spring"
equation "cop_canale_fondo_raggio_esterno = 40.0 mm" comment "Fondo liscio pista cavi tipo clock-spring"
equation "cop_canale_fondo_quota = 20.0 mm" comment "Quota locale fondo pista cavi"
equation "cop_canale_fondo_spessore = 3.0 mm" comment "Fondo strutturale pista cavi"
equation "cop_canale_parete_spessore = 1.5 mm" comment "Pareti lisce pista cavi"
equation "cop_canale_altezza_libera = 7.0 mm" comment "Altezza libera pista cavi"
equation "stepper_corpo_diametro = 28.0 mm" comment "Riferimento stepper"
equation "stepper_corpo_altezza = 20.0 mm" comment "Riferimento stepper"
equation "stepper_albero_diametro = 5.0 mm" comment "Riferimento stepper"
equation "stepper_albero_lunghezza = 9.0 mm" comment "Riferimento stepper"
equation "stepper_interasse_fori = 35.0 mm" comment "Fissaggio stepper"
equation "stepper_foro_fissaggio = 4.2 mm" comment "Fissaggio stepper"
equation "torre_base_diametro = 70.0 mm" comment "Adattatore rotante"
equation "torre_base_spessore = 6.0 mm" comment "Adattatore rotante"
equation "torre_fissa_larghezza = 80.0 mm" comment "Parte fissa torretta"
equation "torre_fissa_lunghezza = 70.0 mm" comment "Parte fissa torretta"
equation "torre_fissa_altezza = 50.0 mm" comment "Parte fissa torretta"
equation "torre_parete_spessore = 4.0 mm" comment "Parte fissa torretta"
equation "torre_perno_quota = 32.0 mm" comment "Asse elevazione"
equation "servo_corpo_lunghezza = 22.7 mm" comment "TowerPro SG90"
equation "servo_corpo_larghezza = 12.2 mm" comment "TowerPro SG90"
equation "servo_corpo_altezza = 27.0 mm" comment "TowerPro SG90"
equation "servo_ingombro_con_uscita = 30.3 mm" comment "TowerPro SG90"
equation "servo_alette_lunghezza_totale = 32.3 mm" comment "TowerPro SG90"
equation "servo_asse_da_estremita = 17.0 mm" comment "TowerPro SG90"
equation "servo_albero_sporgenza = 3.3 mm" comment "TowerPro SG90"
equation "servo_perno_diametro = 6.0 mm" comment "Perni servo coassiali"
equation "servo_gioco_inserimento = 0.5 mm" comment "Slitta servo"
equation "servo_supporto_parete = 2.5 mm" comment "Slitta servo"
equation "servo_supporto_ripiano = 2.5 mm" comment "Slitta servo"
equation "servo_barretta_spessore = 3.0 mm" comment "Chiusura removibile servo"
equation "servo_barretta_sovrapposizione = 3.0 mm" comment "Chiusura removibile servo"
equation "servo_foro_M2_5 = 2.7 mm" comment "Chiusura removibile servo"
equation "servo_preforo_M2_5 = 2.2 mm" comment "Slitta servo"
equation "servo_cavo_larghezza = 4.0 mm" comment "Cavo piatto SG90"
equation "servo_cavo_spessore = 1.0 mm" comment "Cavo piatto SG90"
equation "servo_uscita_cavo_larghezza = 5.0 mm" comment "Slitta SG90"
equation "servo_uscita_cavo_profondita = 2.0 mm" comment "Slitta SG90"
equation "servo_connettore_larghezza = 7.0 mm" comment "Connettore SG90"
equation "servo_connettore_spessore = 3.0 mm" comment "Connettore SG90"
equation "passaggio_comune_larghezza = 8.0 mm" comment "Passaggio connettori SG90"
equation "passaggio_comune_lunghezza = 6.0 mm" comment "Passaggio connettori SG90"
equation "passaggio_arco_raggio = 28.0 mm" comment "Guida cavi azimut"
equation "passaggio_arco_larghezza = 8.0 mm" comment "Guida cavi azimut"
equation "cannone_connettore_larghezza = 5.0 mm" comment "Connettore cannone"
equation "cannone_connettore_spessore = 3.0 mm" comment "Connettore cannone"
equation "cannone_passaggio_mobile_larghezza = 6.0 mm" comment "Passaggio sotto culla"
equation "cannone_passaggio_mobile_lunghezza = 4.0 mm" comment "Passaggio sotto culla"
equation "pcb_cannone_lunghezza = 50.0 mm" comment "PCB mobile cannone"
equation "pcb_cannone_larghezza = 50.0 mm" comment "PCB mobile cannone"
equation "pcb_cannone_spessore = 2.0 mm" comment "PCB mobile cannone"
equation "pcb_cannone_foro = 3.5 mm" comment "Fori PCB cannone"
equation "pcb_cannone_foro_bordo_x = 5.0 mm" comment "Fori PCB cannone"
equation "pcb_cannone_foro_bordo_y = 5.0 mm" comment "Fori PCB cannone"
equation "solenoide_diametro = 20.0 mm" comment "Zona solenoide"
equation "solenoide_lunghezza = 25.0 mm" comment "Zona solenoide"
equation "canna_diametro_esterno = 10.0 mm" comment "Canna tubolare"
equation "canna_diametro_interno = 8.0 mm" comment "Canna tubolare"
equation "canna_parete = 1.0 mm" comment "Canna tubolare"
equation "canna_sporgenza = 46.0 mm" comment "Canna tubolare"
equation "modulo_cannone_altezza = 23.0 mm" comment "Modulo mobile"
equation "cannone_elevazione_min = -10.0 deg" comment "Limite proposto asse elevazione"
equation "cannone_elevazione_max = 35.0 deg" comment "Limite proposto asse elevazione"
equation "passaggio_arco_angolo_iniziale = 0.0 deg" comment "Inizio guida cavi di azimut"
equation "passaggio_arco_corsa = 360.0 deg" comment "Corsa totale guida cavi di azimut"
equation "torretta_azimut_min = -180.0 deg" comment "Limite software e giunto Fusion"
equation "torretta_azimut_max = 180.0 deg" comment "Limite software e giunto Fusion"
equation "d219 = cop_parete_altezza"
equation "d221 = cop_tetto_spessore"
equation "d239 = cop_parete_altezza"
equation "d241 = cop_tetto_spessore"
equation "d243 = cop_tetto_spessore"
equation "d245 = cop_tetto_spessore"
equation "d255 = cop_canale_fondo_spessore"
equation "d257 = cop_canale_fondo_spessore"
equation "d259 = cop_tetto_spessore"
equation "d263 = stepper_corpo_altezza"
equation "d271 = stepper_albero_lunghezza"
equation "d275 = torre_base_spessore"
equation "d277 = torre_base_spessore"
equation "d279 = torre_base_spessore"
equation "d283 = torre_base_spessore"
equation "d287 = torre_base_spessore"
equation "d291 = torre_base_spessore"
equation "d295 = torre_base_spessore"
equation "d299 = torre_base_spessore"
equation "d397 = servo_corpo_altezza"
equation "d401 = servo_albero_sporgenza"
equation "d405 = servo_corpo_altezza"
equation "d409 = servo_albero_sporgenza"
equation "d413 = servo_barretta_spessore"
equation "d417 = servo_barretta_spessore"
equation "d421 = servo_barretta_spessore"
equation "d425 = servo_barretta_spessore"
equation "d429 = servo_barretta_spessore"
equation "d433 = servo_barretta_spessore"
equation "d437 = servo_barretta_spessore"
equation "d441 = servo_barretta_spessore"
equation "d483 = pcb_cannone_spessore"
equation "d485 = pcb_cannone_spessore"
equation "d487 = pcb_cannone_spessore"
equation "d489 = pcb_cannone_spessore"
equation "d491 = pcb_cannone_spessore"
equation "d499 = solenoide_lunghezza"
equation "d503 = solenoide_lunghezza"
equation "d507 = canna_sporgenza"
equation "d511 = canna_sporgenza"
equation "guscio_torretta_parete = 2.5 mm" comment "Gusci removibili torretta"
equation "guscio_torretta_gioco = 0.5 mm" comment "Gioco attorno a telaio, servo e modulo mobile"
equation "guscio_cannone_foro_canna = 11.0 mm" comment "Passaggio canna nel guscio mobile"
named bodies: "Piano_inferiore_colonnine_M3_supporto_batteria_integrato", "Piano_superiore", "Guscio_laterale_continuo_166x176_Z0_Z76", "Tetto_removibile_canale_clock_spring_supporto_stepper_boss_M3", "Corpo_stepper", "Piastra_adattatore_rotante", "Base_parte_fissa", "Corpo_SG90_Sinistro", "Corpo_SG90_Destro", "Barretta_Sinistra_01", "Barretta_Sinistra_02", "Barretta_Destra_01", "Barretta_Destra_02", "Piastra_culla_mobile", "PCB_modulo_cannone_50x50", "Appoggio_solenoide_su_PCB", "Corpo_solenoide_riferimento", "Canna_tubolare_esterna", "Parete_posteriore_guscio_torretta", "Parete_esterna_carter_Sinistro", "Parete_esterna_carter_Destro", "Parete_mobile_Ovest", "Canna_tubolare_esterna (1)"
